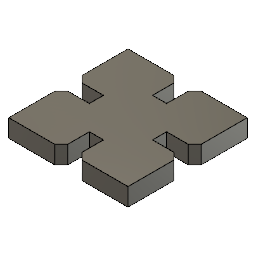
parametricv11 (Autodesk Fusion 360 design; units mm, degrees)
Autodesk Fusion 360 part; units mm, degrees
sketch "Sketch1" plane through (0, 0, 0) normal (0, 1, 0) x (1, 0, 0)
  line L0 (13.6189, 1.605) -> (13.6189, 13.6189)
  line L1 (-13.6189, 13.6189) -> (-13.6189, 1.605)
  line L2 (13.6189, -1.605) -> (13.6189, -13.6189)
  line L3 (-13.6189, -13.6189) -> (-13.6189, -1.605)
  line L4 (1.605, 7.1989) -> (1.605, 13.6189)
  line L5 (0, 0) -> (2.5, 0)
  line L6 (7.1989, 1.605) -> (13.6189, 1.605)
  line L7 (7.1989, -1.605) -> (13.6189, -1.605)
  line L8 (13.6189, 13.6189) -> (1.605, 13.6189)
  line L9 (-1.605, 13.6189) -> (-13.6189, 13.6189)
  line L10 (-13.6189, 13.6189) -> (0, 0)
  line L11 (0, 0) -> (13.6189, 13.6189)
  line L12 (-13.6189, -13.6189) -> (0, 0)
  line L13 (0, 0) -> (13.6189, -13.6189)
  line L14 (7.1989, 1.605) -> (7.1989, -1.605)
  line L15 (-7.1989, -1.605) -> (-13.6189, -1.605)
  line L16 (-7.1989, 1.605) -> (-7.1989, -1.605)
  line L17 (-7.1989, 1.605) -> (-13.6189, 1.605)
  line L18 (-1.605, 7.1989) -> (-1.605, 13.6189)
  line L19 (1.605, 7.1989) -> (-1.605, 7.1989)
  line L20 (-1.605, -7.1989) -> (-1.605, -13.6189)
  line L21 (1.605, -7.1989) -> (1.605, -13.6189)
  line L22 (1.605, -7.1989) -> (-1.605, -7.1989)
  line L23 (13.6189, -13.6189) -> (1.605, -13.6189)
  line L24 (-1.605, -13.6189) -> (-13.6189, -13.6189)
  line L25 (81.6508, 319732.5239) -> (6.33, 319732.5239)
  line L26 (81.6508, 319732.5239) -> (102.864, 319753.7371)
  line L27 (92.864, 319735.0239) -> (102.864, 319735.0239)
  line L28 (102.864, 319753.7371) -> (84.1508, 319753.7371)
  line L29 (92.864, 319730.0239) -> (102.864, 319730.0239)
  line L30 (102.864, 319735.0239) -> (102.864, 319753.7371)
  line L31 (60.4376, 319753.7371) -> (60.4376, 319735.0239)
  line L32 (60.4376, 319711.3107) -> (60.4376, 319730.0239)
  line L33 (84.1508, 319743.7371) -> (84.1508, 319753.7371)
  line L34 (60.4376, 319711.3107) -> (81.6508, 319732.5239)
  line L35 (102.864, 319730.0239) -> (102.864, 319711.3107)
  line L36 (60.4376, 319753.7371) -> (81.6508, 319732.5239)
  line L37 (84.1508, 319721.3107) -> (79.1508, 319721.3107)
  line L38 (84.1508, 319721.3107) -> (84.1508, 319711.3107)
  line L39 (79.1508, 319721.3107) -> (79.1508, 319711.3107)
  line L40 (84.1508, 319743.7371) -> (79.1508, 319743.7371)
  line L41 (79.1508, 319743.7371) -> (79.1508, 319753.7371)
  line L42 (92.864, 319735.0239) -> (92.864, 319730.0239)
  line L43 (81.6508, 319732.5239) -> (102.864, 319711.3107)
  line L44 (79.1508, 319753.7371) -> (60.4376, 319753.7371)
  line L45 (79.1508, 319711.3107) -> (60.4376, 319711.3107)
  line L46 (70.4376, 319730.0239) -> (60.4376, 319730.0239)
  line L47 (70.4376, 319735.0239) -> (70.4376, 319730.0239)
  line L48 (70.4376, 319735.0239) -> (60.4376, 319735.0239)
  line L49 (102.864, 319711.3107) -> (84.1508, 319711.3107)
  dimension "d9" = 19.26
  dimension "d15" = 6.42
  dimension "d60" = 30
  dimension "d61" = 10
  dimension "d62" = 5
  dimension "d69" = 3.21
  measures "d9" distance of L5.start
extrude "Extrude1" add sketch "Sketch1" along normal blind 4.1 contours L0 L2 L6 L7 L11 L13 L14 | L4 L8 L9 L10 L11 L18 L19 | L1 L3 L10 L12 L15 L16 L17 | L12 L13 L20 L21 L22 L23 L24
chamfer "Chamfer1" distance 1.5 angle 45 8 edges at (-13.6189, 2.05, 1.605) (-13.6189, 2.05, -1.605) (-1.605, 2.05, -13.6189) (1.605, 2.05, -13.6189) (13.6189, 2.05, -1.605) (13.6189, 2.05, 1.605) (1.605, 2.05, 13.6189) (-1.605, 2.05, 13.6189) measured on face at (-9.3389, 1.3667, 1.605) measured on face at (-13.6189, 1.3667, -9.6143) measured on face at (-1.605, 2.7333, -11.4789) measured on face at (9.6143, 1.3667, -13.6189) measured on face at (9.3389, 1.3667, -1.605) measured on face at (13.6189, 1.3667, 5.6096) measured on face at (1.605, 1.3667, 9.3389) measured on face at (-5.6096, 1.3667, 13.6189)
equation "d9 = THICKNESS * 6"
equation "d15 = THICKNESS * 2"
equation "SLOT = 10 mm"
equation "d60 = SLOT * 3"
equation "d61 = SLOT"
equation "d62 = SLOT / 2"
equation "d69 = THICKNESS"
equation "THICKNESS = 3.21 mm"
